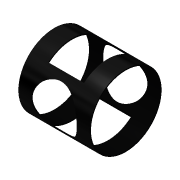
# Autodesk Inventor part: scatterBlock
Saved by Autodesk Inventor 2015 SP1 (Build 190203100, 203)
## iProperties
Created: 2016-10-04
Part Number: scatterBlock
Material: Generic
Document SubType Name: Modeling
Designer: I Rabey
Density: 1 g/cm^3
Appearance: Default
Author: I Rabey
Autodesk Inventor part; units mm, degrees
ref_plane "YZ Plane" through (0, 0, 0) normal (1, 0, 0) x (0, 1, 0)
sketch "Sketch1" plane through (0, 0, 0) normal (1, 0, 0) x (0, 1, 0)
  circle A0 centre (0.8255, 0) radius 29.2
  circle A1 centre (0.8255, 0) radius 30.2
  point P0 (0, 0)
  dimension "d0" = 58.4
  dimension "d1" = 60.4
  constraints: 2 centre point, 1 coincident
  measures "d0" diameter of A0
  measures "d1" diameter of A1
extrude "Extrusion1" add sketch "Sketch1" along normal mid plane 60
ref_plane "Work Plane1" through (0, 31.0255, 0) normal (0, 1, 0) x (-1, 0, 0)
sketch "Sketch2" plane through (0, 31.0255, 0) normal (0, 1, 0) x (-1, 0, 0)
  line L0 (-15, -20) -> (15, -20)
  line L1 (15, -20) -> (15, 20)
  line L2 (15, 20) -> (-15, 20)
  line L3 (-15, 20) -> (-15, -20)
  line L4 (-15, -20) -> (15, 20) construction
  line L5 (15, -20) -> (-15, 20) construction
  point P0 (0, 0)
  dimension "d4" = 30
  dimension "d5" = 40
  constraints: 12 end point, 2 midpoint, 2 parallel, 1 horizontal, 1 perpendicular
  measures "d4" distance of L2.end L1.end
  measures "d5" distance of L1.end L0.end
extrude "Extrusion2" cut sketch "Sketch2" against normal blind 80
ref_plane "Work Plane2" through (0, 0.8255, 30.2) normal (0, 0, 1) x (1, 0, 0)
sketch "Sketch3" plane through (0, 0.8255, 30.2) normal (0, 0, 1) x (1, 0, 0)
  circle A0 centre (0, -0.8255) radius 19.05
  dimension "d8" = 38.1
  constraints: 1 centre point, 1 coincident
  measures "d8" diameter of A0
extrude "Extrusion3" cut sketch "Sketch3" against normal blind 80
body "Solid1"
